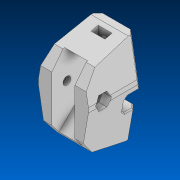
# Autodesk Inventor part: y-idler-V2
Saved by Autodesk Inventor 2021 (Build 250183000, 183)
## iProperties
Created: 2021-03-09
Part Number: y-idler-V2
Material: Generic
Document SubType Name: Modeling
Designer: Alex
Density: 1 g/cm^3
Appearance: Default
Author: Alex
## iProperties of the stored document _3DPrint.ipt
Created: 2021-03-16
Part Number: _3DPrint
Material: Generic
Document SubType Name: Modeling
Designer: Alex
Density: 1 g/cm^3
Appearance: Default
Author: Alex
Autodesk Inventor part; units mm, degrees
sketch "Sketch1" plane through (0, 0, 0) normal (0, 0, 1) x (1, 0, 0)
  line L0 (-8.0906, 16.5) -> (8.0906, 16.5)
  line L1 (8.0906, 16.5) -> (11, 0)
  line L2 (11, 0) -> (6.8563, -23.5)
  line L3 (6.8563, -23.5) -> (-6.8563, -23.5)
  line L4 (-6.8563, -23.5) -> (-11, 0)
  line L5 (-11, 0) -> (-8.0906, 16.5)
  line L6 (0, 0) -> (0, 30.665) construction
  line L7 (0, 0) -> (39.242, 0) construction
  line L8 (-10.8237, 1) -> (-10.8237, -1)
  line L9 (10.8237, 1) -> (10.8237, -1)
  dimension "d0" = 80
  dimension "d1" = 100
  dimension "d2" = 16.5
  dimension "d3" = 40
  dimension "d4" = 22
  dimension "d5" = 2
  constraints: 20 end point, 5 symmetric about line, 3 point on line, 2 horizontal, 2 vertical, 1 parallel
  measures "d0" angle of L7 L1
  measures "d1" angle of L7 L2
  measures "d2" distance between parallel lines of L7 L0
  measures "d3" distance between parallel lines of L3 L0
  measures "d4" distance of L1.end L4.end
  measures "d5" distance of L8.start L8.end
extrude "Extrusion1" add sketch "Sketch1" along normal blind 23 contours L0 L1 L9 L2 L3 L4 L8 L5
ref_plane "Work Plane1" through (0, 0, 0) normal (1, 0, 0) x (0, 1, 0)
sketch "Sketch2" plane through (0, 0, 0) normal (1, 0, 0) x (0, 1, 0)
  circle A0 centre (0, 16.5) radius 1.7
  line L0 (0, 0) -> (0, 23) construction
  line L1 (1, 23) -> (-1, 23) projected
  arc A1 (-10, 16.5) -> (10, 16.5) centre (0, 16.5) ccw
  line L2 (-10, 16.5) -> (-10, 23)
  line L3 (-1, 23) -> (-23.5, 23) projected
  line L4 (10, 16.5) -> (10, 23)
  line L5 (8.1915, 10.7642) -> (19.7547, 27.2782)
  line L6 (-7.0711, 9.4289) -> (-20.6421, 23)
  line L7 (-23.5, 0) -> (-23.5, 23) projected
  line L8 (-23.5, 23) -> (-23.5, 0)
  line L9 (16.5, 0) -> (1, 0) projected
  line L10 (-23.5, 0) -> (16.5, 0)
  line L11 (16.5, 0) -> (16.5, 23) projected
  line L12 (16.5, 0) -> (16.5, 23)
  line L13 (16.5, 23) -> (-23.5, 23)
  line L14 (-23.5, 0) -> (-23.5, 3)
  line L15 (16.5, 0) -> (16.5, 3)
  line L16 (16.5, 23) -> (1, 23) projected
  line L17 (-23.5, 3) -> (-19.25, 20)
  line L18 (-19.25, 20) -> (-18.5, 23)
  line L19 (16.5, 3) -> (12.25, 20)
  line L20 (12.25, 20) -> (11.5, 23)
  line L21 (-23.5, 0) -> (-1, 0) projected
  line L22 (-10.5, 0) -> (-10.5, 5.5)
  line L23 (-10.5, 5.5) -> (-9.25, 6.75)
  line L24 (-9.25, 6.75) -> (-4.75, 6.75)
  line L25 (-4.75, 6.75) -> (-3.5, 5.5)
  line L26 (-3.5, 5.5) -> (-3.5, 0)
  line L27 (-7, 6.75) -> (-7, 0) construction
  point P0 (-1.75, 2.75)
  point P1 (16.5, 22.63)
  dimension "d9" = 3.4
  dimension "d10" = 16.5
  dimension "d11" = 20
  dimension "d12" = 35
  dimension "d13" = 45
  dimension "d14" = 3
  dimension "d18" = 4.25
  dimension "d19" = 17
  dimension "d25" = 6.75
  dimension "d26" = 7
  dimension "d27" = 45
  dimension "d28" = 45
  dimension "d29" = 7
  dimension "d30" = 1.25
  constraints: 42 end point, 12 point on line, 7 perpendicular, 6 equal length, 4 point on circle, 3 tangent, 2 centre point, 2 midpoint, 1 coincident, 1 vertical, 1 other
  measures "d9" diameter of A0
  measures "d10" distance of A0.centre L0.start
  measures "d11" distance between parallel lines of L4 L2
  measures "d12" angle of L5 L4
  measures "d13" angle of L2 L6
  measures "d14" distance of L7.start L14.end
  measures "d18" distance from line of L19.end L15
  measures "d19" vertical distance of L19.end L15.end
  measures "d25" distance between parallel lines of L24 L10
  measures "d26" distance between parallel lines of L26 L22
  measures "d27" angle of L22 L23
  measures "d28" angle of L26 L25
  measures "d29" distance between parallel lines of L27 L0
  measures "d30" horizontal distance of L22.end L23.end
extrude "Extrusion2" cut sketch "Sketch2" against normal through all both and the other way through all contours L13 L11 L5 L19 L20 | L18 L6 L3 | L6 L18 L17 L7 L3 | L5 L11 L19
extrude "Extrusion3" cut sketch "Sketch2" against normal mid plane 10 contours A0 | L13 L4 A1 L2 L3 L1 | L13 L20 L19 L5 A1 L4 | L2 A1 L6 L18 L3 | L13 L11 L5 L19 L20 | L18 L6 L3
extrude "Extrusion4" cut sketch "Sketch2" along normal through all both and the other way through all contours A0 | L22 L23 L24 L25 L26 L10
chamfer "Chamfer1" distance 5 angle 45 3 edges at (-6.369, -18.5, 23) (-6.9861, 11.5, 23) (6.9861, 11.5, 23)
ref_plane "Work Plane2" through (0, 0, 8) normal (0, 0, -1) x (-1, 0, 0)
sketch "Sketch4" plane through (0, 0, 8) normal (0, 0, -1) x (-1, 0, 0)
  circle A0 centre (0, -18) radius 1.7
  circle A1 centre (0, 12) radius 1.7
  line L0 (-6.8563, -23.5) -> (6.8563, -23.5) projected
  line L1 (3, -23.5) -> (-3, -23.5)
  line L2 (-3, -23.5) -> (-3, -14.5)
  line L3 (-3, -14.5) -> (3, -14.5)
  line L4 (3, -14.5) -> (3, -23.5)
  line L5 (8.0906, 16.5) -> (-8.0906, 16.5) projected
  line L6 (3, 16.5) -> (-3, 16.5)
  line L7 (-3, 16.5) -> (-3, 8.5)
  line L8 (-3, 8.5) -> (3, 8.5)
  line L9 (3, 8.5) -> (3, 16.5)
  line L10 (0, -31.5) -> (0, 24.5) projected
  point P0 (0, 0)
  dimension "d41" = 18
  dimension "d42" = 12
  dimension "d43" = 3.4
  dimension "d44" = 3.5
  dimension "d45" = 3.5
  dimension "d46" = 6
  dimension "d47" = 6
  constraints: 16 end point, 4 parallel, 4 point on line, 2 centre point, 2 horizontal, 2 perpendicular, 1 equal radius, 2 other
  measures "d41" distance of A0.centre point (0, 0)
  measures "d42" distance of A1.centre point (0, 0)
  measures "d43" diameter of A1
  measures "d44" distance from line of L3 A0.centre
  measures "d45" distance from line of L8 A1.centre
  measures "d46" distance of L6.start L6.end
  measures "d47" distance between parallel lines of L2 L4
extrude "Extrusion5" cut sketch "Sketch4" along normal blind 10 and the other way blind 4 contours A0 L10 | L10 A0 | A1 L10 | L10 A1
extrude "Extrusion6" cut sketch "Sketch4" along normal blind 3
chamfer "Chamfer2" distance 2 angle 45 4 edges at (-9.4571, 8.75, 0) (-8.0024, -17, 0) (8.0024, -17, 0) (9.4571, 8.75, 0)
chamfer "Chamfer3" distance 0.5 angle 45 16 edges at (0, -3.5, 0) (-9.9846, -3.5, 0.3922) (-10.3829, -3.5, 3.1422) (9.9846, -3.5, 0.3922) (10.3829, -3.5, 3.1422) (0, -10.5, 0) (8.1331, -10.5, 1) (9.1486, -10.5, 3.75) (-8.1331, -10.5, 1) (-9.1486, -10.5, 3.75) (-10.2727, -4.125, 6.125) (-9.7657, -7, 6.75) (-9.2588, -9.875, 6.125) (9.2588, -9.875, 6.125) (9.7657, -7, 6.75) (10.2727, -4.125, 6.125)
ref_plane "Work Plane3" through (7, 0, 0) normal (1, 0, 0) x (0, 1, 0)
sketch "Sketch5" plane through (7, 0, 0) normal (1, 0, 0) x (0, 1, 0)
  arc A0 (-1, 17.8748) -> (-1, 15.1252) centre (0, 16.5) ccw projected
  arc A1 (1, 17.8748) -> (-1, 17.8748) centre (0, 16.5) ccw projected
  line L0 (3, 18.2321) -> (3, 14.7679)
  line L1 (3, 14.7679) -> (0, 13.0359)
  line L2 (0, 13.0359) -> (-3, 14.7679)
  line L3 (-3, 14.7679) -> (-3, 18.2321)
  line L4 (-3, 18.2321) -> (0, 19.9641)
  line L5 (0, 19.9641) -> (3, 18.2321)
  point P0 (0, 0)
  dimension "d61" = 6
  constraints: 12 end point, 1 coincident, 1 vertical, 13 other
  measures "d61" distance between parallel lines of L0 L3
extrude "Extrusion7" cut sketch "Sketch5" along normal through all
ref_plane "Work Plane4" through (-7, 0, 0) normal (1, 0, 0) x (0, 1, 0)
sketch "Sketch6" plane through (-7, 0, 0) normal (1, 0, 0) x (0, 1, 0)
  arc A0 (-1, 17.8748) -> (-1, 15.1252) centre (0, 16.5) ccw projected
  circle A1 centre (0, 16.5) radius 1.7 projected
  circle A2 centre (0, 16.5) radius 3
  point P0 (0, 0)
  constraints: 1 centre point, 1 coincident
extrude "Extrusion8" cut sketch "Sketch6" against normal through all contours A1 A0 | A2
equation "\"d45\" = d44"
equation "\"d47\" = d46"
body "Solid1"
